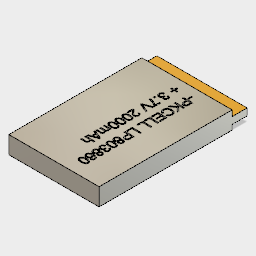
07_2000mAh_Battery v1 v1 (Autodesk Fusion 360 design; units mm, degrees)
Autodesk Fusion 360 part; units mm, degrees
sketch "Sketch1" plane through (0, 0, 0) normal (0, 0, 1) x (1, 0, 0)
  line L0 (18, -3.5) -> (-18, -3.5)
  line L1 (-18, -3.5) -> (-18, 3.5)
  line L2 (-18, 3.5) -> (18, 3.5)
  line L3 (18, 3.5) -> (18, -3.5)
  line L4 (18, -3.5) -> (-18, 3.5) construction
  line L5 (-18, -3.5) -> (18, 3.5) construction
  dimension "d1" = 36
  dimension "d2" = 7
  measures "d1" distance of L1.end L2.end
  measures "d2" distance of L0.end L1.end
extrude "Extrude1" add sketch "Sketch1" along normal blind 53
sketch "Sketch2" plane through (0, 0, 0) normal (0, 0, -1) x (-1, 0, 0)
  line L0 (18, 3.5) -> (-18, 3.5)
  line L1 (-18, 3.5) -> (-18, -3.5)
  line L2 (-18, -3.5) -> (18, -3.5)
  line L3 (18, -3.5) -> (18, 3.5)
  line L4 (18, 1.1901) -> (-18, 1.1901)
  line L5 (-18, 1.1901) -> (-18, -1.5599)
  line L6 (-18, -1.5599) -> (18, -1.5599)
  line L7 (18, -1.5599) -> (18, 1.1901)
  dimension "d5" = 2.75
  measures "d5" distance of L4.start L6.end
extrude "Extrude2" add sketch "Sketch2" along normal blind 6 contours L1 L3 L4 L5 L6 L7
sketch "Sketch3" plane through (0, 3.5, 0) normal (0, 1, 0) x (-1, 0, 0)
  line L0 (-18, 0) -> (18, 0)
  line L1 (18, 0) -> (18, 53)
  line L2 (18, 53) -> (-18, 53)
  line L3 (-18, 53) -> (-18, 0)
  line L4 (-4.035, 3.5) -> (-4.035, 48.1338) construction
  line L5 (-4.035, 48.1338) -> (-9.035, 48.1338) construction
  line L6 (-9.035, 48.1338) -> (-9.035, 3.5) construction
  line L7 (-9.035, 3.5) -> (-4.035, 3.5) construction
  line L8 (2.2527, 3.5) -> (2.2527, 40.27) construction
  line L9 (2.2527, 40.27) -> (-2.7473, 40.27) construction
  line L10 (-2.7473, 40.27) -> (-2.7473, 3.5) construction
  line L11 (-2.7473, 3.5) -> (2.2527, 3.5) construction
  text T0 "-PKCELL LP803860" font "Arial" height 5 align ink ink in box 0 x 0 at (-4.055, 3.51) x (0, 1) y (-1, 0) spacing 1 height is em
  text T1 "+ 3.7V 2000mAh" font "Arial" height 5 align ink ink in box 0 x 0 at (2.2327, 3.51) x (0, 1) y (-1, 0) spacing 1 height is em
extrude "Extrude3" cut sketch "Sketch3" against normal blind 1 text T0 T1
